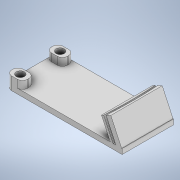
# Autodesk Inventor part: Sostenedor MQ
Saved by Autodesk Inventor 2020.3 (Build 243373000, 373)
## iProperties
Created: 2021-05-13
Part Number: Sostenedor MQ
Material: Generic
Document SubType Name: Modeling
Designer: juanp
Density: 1 g/cm^3
Appearance: Default
Author: juanp
Autodesk Inventor part; units mm, degrees
ref_plane "YZ Plane" through (0, 0, 0) normal (1, 0, 0) x (0, 1, 0)
ref_plane "XZ Plane" through (0, 0, 0) normal (0, 1, 0) x (-1, 0, 0)
ref_plane "XY Plane" through (0, 0, 0) normal (0, 0, 1) x (1, 0, 0)
sketch "Sketch1" plane through (0, 0, 0) normal (0, 1, 0) x (-1, 0, 0)
  line L0 (0, 0) -> (45, 0)
  line L1 (45, 0) -> (45, -20)
  line L2 (45, -20) -> (0, -20)
  line L3 (0, -20) -> (0, 0)
  circle A0 centre (41.875, -2.25) radius 1.6
  circle A1 centre (41.875, -17.75) radius 1.6
  line L4 (41.875, -2.25) -> (41.875, -17.75) construction
  line L5 (41.875, -2.25) -> (41.875, 0) construction
  line L6 (41.875, -17.75) -> (41.875, -20) construction
  dimension "d0" = 45
  dimension "d1" = 20
  dimension "d3" = 3.125
  dimension "d4" = 3.2
  dimension "d5" = 15.5
  constraints: 14 end point, 3 point on line, 2 centre point, 2 parallel, 2 perpendicular, 1 collinear, 1 equal radius, 1 horizontal, 1 vertical
  measures "d0" distance of L1.end L2.end
  measures "d1" distance of L2.end L0.start
  measures "d3" distance between parallel lines of L1 L4
  measures "d4" diameter of A0
  measures "d5" distance of L4.start L4.end
extrude "Extrusion1" add sketch "Sketch1" along normal blind 2
sketch "Sketch2" plane through (0, 2, 0) normal (0, 1, 0) x (1, 0, 0)
  line L0 (-45, 0) -> (0, 0) projected
  line L1 (-45, 0) -> (-38.75, 0)
  line L2 (-38.75, 0) -> (-38.75, 4.5)
  line L3 (-38.75, 4.5) -> (-45, 4.5)
  line L4 (-45, 4.5) -> (-45, 0)
  line L5 (0, 20) -> (-45, 20) projected
  line L6 (-45, 20) -> (-38.75, 20)
  line L7 (-38.75, 20) -> (-38.75, 15.5)
  line L8 (-38.75, 15.5) -> (-45, 15.5)
  line L9 (-45, 15.5) -> (-45, 20)
  circle A0 centre (-41.875, 2.25) radius 1.6 projected
  line L10 (-41.875, 0) -> (-41.875, 2.25) construction
  line L11 (-41.875, 2.25) -> (-41.875, 4.5) construction
  line L12 (-41.875, 2.25) -> (-45, 2.25) construction
  line L13 (-45, 20) -> (-45, 0) projected
  line L14 (-41.875, 2.25) -> (-38.75, 2.25) construction
  circle A1 centre (-41.875, 17.75) radius 1.6 projected
  constraints: 24 end point, 4 equal length, 4 parallel, 3 midpoint, 3 perpendicular, 2 horizontal, 2 vertical, 1 point on line
extrude "Extrusion2" add sketch "Sketch2" along normal blind 3
fillet "Fillet1" radius 2 8 edges at (-38.75, 3.5, -15.5) (-38.75, 3.5, -4.5) (-38.75, 3.5, 0) (-45, 3.5, -4.5) (-45, 2.5, 0) (-38.75, 3.5, -20) (-45, 3.5, -15.5) (-45, 2.5, -20)
ref_plane "Work Plane2" through (-4.2262, 11.0631, 0) normal (0.4226183, -0.9063078, 0) x (0, 0, -1)
ref_plane "Work Plane1" through (0, 2, 0) normal (0.4226183, -0.9063078, 0) x (0, 0, -1)
sketch "Sketch3" plane through (-4.2262, 11.0631, 0) normal (0.4226183, -0.9063078, 0) x (0, 0, -1)
  line L0 (0, -36.932) -> (0, 0) projected
  line L1 (20, 0) -> (20, -36.932) projected
  arc A0 (20, -3.1957) -> (0, -3.1957) centre (10, -76.5169) ccw
  line L2 (20, -0.8452) -> (20, 0) projected
  arc A1 (20, -2.1866) -> (0, -2.1866) centre (10, -76.5169) ccw
  line L3 (0, 0) -> (20, 0) projected
  line L4 (10, 0) -> (10, -76.5169) construction
  line L5 (0, -4.1957) -> (20, -4.1957)
  line L6 (20, -4.1957) -> (20, -0.1866)
  line L7 (20, -0.1866) -> (0, -0.1866)
  line L8 (0, -0.1866) -> (0, -4.1957)
  point P0 (0, -0.8452)
  point P1 (20, -0.1866)
  point P2 (0, -0.1866)
  dimension "d13" = 74
  dimension "d14" = 75
  dimension "d15" = 1
  dimension "d16" = 2
  constraints: 10 end point, 6 point on line, 4 point on circle, 2 centre point, 2 parallel, 1 coincident, 1 horizontal, 1 midpoint, 1 perpendicular, 1 vertical
  measures "d13" radius of A0
  measures "d14" radius of A1
  measures "d15" distance of L5.end A0.start
  measures "d16" distance of A1.start L6.end
extrude "Extrusion3" add sketch "Sketch3" along normal up to next contours L0 A0 L1 L5 | L0 L7 L1 A1
body "Solid1"
